Autodesk Fusion 360 part; units mm, degrees
(part 6 of 8)
  spline S170 degree 5 poles (-253.8232, -300.3539) (-253.7673, -300.4279) (-253.6554, -300.5759) (-253.4871, -300.7975) (-253.2622, -301.0921) (-252.9798, -301.4591) (-252.6964, -301.8248) (-252.4118, -302.1892) (-252.1261, -302.5523) (-251.8392, -302.914) (-251.5513, -303.2744) (-251.2621, -303.6334) (-250.9719, -303.9911) (-250.6805, -304.3474) (-250.388, -304.7023) (-250.0943, -305.0558) (-249.7994, -305.4078) (-249.5034, -305.7584) (-249.2062, -306.1076) (-248.9079, -306.4553) (-248.6083, -306.8015) (-248.3076, -307.1462) (-248.0057, -307.4895) (-247.7026, -307.8312) (-247.3983, -308.1713) (-247.0928, -308.5099) (-246.7861, -308.8469) (-246.4782, -309.1823) (-246.1691, -309.5161) (-245.8587, -309.8483) (-245.5471, -310.1788) (-245.2342, -310.5077) (-244.9201, -310.8348) (-244.6048, -311.1603) (-244.2881, -311.484) (-243.9702, -311.8059) (-243.651, -312.1261) (-243.3305, -312.4444) (-243.0087, -312.7609) (-242.6855, -313.0755) (-242.361, -313.3882) (-242.0352, -313.699) (-241.7081, -314.0079) (-241.3795, -314.3147) (-241.0496, -314.6196) (-240.7183, -314.9223) (-240.3856, -315.223) (-240.0514, -315.5215) (-239.7157, -315.8178) (-239.3786, -316.1118) (-239.04, -316.4036) (-238.6999, -316.6931) (-238.3583, -316.9802) (-238.0151, -317.2649) (-237.6704, -317.5471) (-237.324, -317.8267) (-236.9759, -318.1036) (-236.626, -318.3775) (-236.2744, -318.6485) (-235.921, -318.9166) (-235.5658, -319.1817) (-235.2088, -319.4439) (-234.85, -319.703) (-234.525, -319.9335) (-234.2708, -320.1107) (-234.0884, -320.236) (-233.9786, -320.3108) (-233.9417, -320.3358) knots -1 -1 -1 -1 -1 -1 -0.98571429 -0.97142857 -0.95714286 -0.94285714 -0.92857143 -0.91428571 -0.9 -0.88571429 -0.87142857 -0.85714286 -0.84285714 -0.82857143 -0.81428571 -0.8 -0.78571429 -0.77142857 -0.75714286 -0.74285714 -0.72857143 -0.71428571 -0.7 -0.68571429 -0.67142857 -0.65714286 -0.64285714 -0.62857143 -0.61428571 -0.6 -0.58571429 -0.57142857 -0.55714286 -0.54285714 -0.52857143 -0.51428571 -0.5 -0.48571429 -0.47142857 -0.45714286 -0.44285714 -0.42857143 -0.41428571 -0.4 -0.38571429 -0.37142857 -0.35714286 -0.34285714 -0.32857143 -0.31428571 -0.3 -0.28571429 -0.27142857 -0.25714286 -0.24285714 -0.22857143 -0.21428571 -0.2 -0.18571429 -0.17142857 -0.15714286 -0.14285714 -0.12857143 -0.11428571 -0.10707295 -0.10707295 -0.10707295 -0.10707295 -0.10707295 -0.10707295
  spline S171 degree 3 poles (-233.3933, -322.3173) (-233.3063, -322.1298) (-233.2568, -321.9271) (-233.2382, -321.5141) (-233.2694, -321.3077) (-233.3956, -320.956) (-233.4764, -320.8087) (-233.681, -320.5447) (-233.8036, -320.4296) (-233.9417, -320.3358) knots 0 0 0 0 0.062015 0.062015 0.12403 0.12403 0.174133 0.174133 0.224236 0.224236 0.224236 0.224236
  arc A86 (-233.3933, -322.3173) -> (-236.8029, -329.9753) centre (11.949, -436.1388) ccw
  spline S172 degree 3 poles (-238.6424, -330.8936) (-238.4416, -330.943) (-238.2332, -330.9527) (-237.8243, -330.8918) (-237.6277, -330.8216) (-237.3067, -330.6303) (-237.1776, -330.5227) (-236.9578, -330.2712) (-236.8684, -330.1289) (-236.8029, -329.9753) knots 0 0 0 0 0.062015 0.062015 0.12403 0.12403 0.174133 0.174133 0.224236 0.224236 0.224236 0.224236
  spline S173 degree 5 poles (-238.6424, -330.8936) (-238.6857, -330.883) (-238.8147, -330.8514) (-239.0299, -330.7997) (-239.3316, -330.7294) (-239.7204, -330.6421) (-240.153, -330.5488) (-240.5867, -330.459) (-241.0214, -330.3724) (-241.4571, -330.2891) (-241.8938, -330.2092) (-242.3315, -330.1325) (-242.7701, -330.059) (-243.2097, -329.9887) (-243.6501, -329.9213) (-244.0913, -329.8569) (-244.5333, -329.7951) (-244.976, -329.7361) (-245.4194, -329.6797) (-245.8635, -329.6259) (-246.3083, -329.5747) (-246.7537, -329.5261) (-247.1998, -329.48) (-247.6465, -329.4363) (-248.0938, -329.3952) (-248.5416, -329.3563) (-248.9901, -329.3199) (-249.4391, -329.2857) (-249.8886, -329.2538) (-250.3386, -329.2242) (-250.7891, -329.1968) (-251.2402, -329.1716) (-251.6917, -329.1486) (-252.1437, -329.1278) (-252.5961, -329.1091) (-253.049, -329.0925) (-253.5023, -329.078) (-253.956, -329.0655) (-254.4101, -329.0551) (-254.8647, -329.0467) (-255.3196, -329.0403) (-255.7749, -329.0359) (-256.2306, -329.0335) (-256.6866, -329.0331) (-257.143, -329.0345) (-257.5997, -329.0379) (-258.0568, -329.0432) (-258.5142, -329.0504) (-258.9719, -329.0595) (-259.4299, -329.0705) (-259.8883, -329.0832) (-260.3469, -329.0979) (-260.8058, -329.1143) (-261.265, -329.1326) (-261.7245, -329.1526) (-262.1843, -329.1745) (-262.6443, -329.1981) (-263.1045, -329.2235) (-263.5651, -329.2507) (-264.0258, -329.2795) (-264.4868, -329.3102) (-264.948, -329.3425) (-265.4094, -329.3765) (-265.8711, -329.4123) (-266.2406, -329.4423) (-266.5178, -329.4655) (-266.7027, -329.4813) (-266.7951, -329.4893) knots 0.10707295 0.10707295 0.10707295 0.10707295 0.10707295 0.10707295 0.11428571 0.12857143 0.14285714 0.15714286 0.17142857 0.18571429 0.2 0.21428571 0.22857143 0.24285714 0.25714286 0.27142857 0.28571429 0.3 0.31428571 0.32857143 0.34285714 0.35714286 0.37142857 0.38571429 0.4 0.41428571 0.42857143 0.44285714 0.45714286 0.47142857 0.48571429 0.5 0.51428571 0.52857143 0.54285714 0.55714286 0.57142857 0.58571429 0.6 0.61428571 0.62857143 0.64285714 0.65714286 0.67142857 0.68571429 0.7 0.71428571 0.72857143 0.74285714 0.75714286 0.77142857 0.78571429 0.8 0.81428571 0.82857143 0.84285714 0.85714286 0.87142857 0.88571429 0.9 0.91428571 0.92857143 0.94285714 0.95714286 0.97142857 0.98571429 1 1 1 1 1 1
  arc A87 (-266.7951, -329.4893) -> (-270.1343, -338.6637) centre (11.949, -436.1388) ccw
  spline S174 degree 5 poles (-270.1343, -338.6637) (-270.0687, -338.7292) (-269.9372, -338.8602) (-269.7398, -339.0562) (-269.476, -339.3167) (-269.1453, -339.6408) (-268.8137, -339.9635) (-268.4812, -340.2847) (-268.1477, -340.6045) (-267.8134, -340.9228) (-267.478, -341.2396) (-267.1418, -341.5549) (-266.8046, -341.8687) (-266.4664, -342.1809) (-266.1273, -342.4917) (-265.7873, -342.8008) (-265.4463, -343.1084) (-265.1044, -343.4144) (-264.7615, -343.7188) (-264.4177, -344.0216) (-264.0729, -344.3228) (-263.7271, -344.6223) (-263.3804, -344.9202) (-263.0327, -345.2164) (-262.684, -345.5108) (-262.3344, -345.8036) (-261.9837, -346.0947) (-261.6321, -346.384) (-261.2796, -346.6715) (-260.926, -346.9573) (-260.5714, -347.2412) (-260.2158, -347.5233) (-259.8592, -347.8035) (-259.5016, -348.0819) (-259.143, -348.3584) (-258.7834, -348.633) (-258.4227, -348.9056) (-258.061, -349.1762) (-257.6983, -349.4448) (-257.3345, -349.7114) (-256.9697, -349.9759) (-256.6038, -350.2384) (-256.2368, -350.4987) (-255.8688, -350.7568) (-255.4997, -351.0128) (-255.1294, -351.2665) (-254.7581, -351.5179) (-254.3856, -351.767) (-254.012, -352.0137) (-253.6372, -352.2579) (-253.2613, -352.4998) (-252.8842, -352.7391) (-252.506, -352.9759) (-252.1265, -353.2101) (-251.7458, -353.4416) (-251.3639, -353.6702) (-250.9807, -353.8959) (-250.5961, -354.1185) (-250.2102, -354.338) (-249.8229, -354.5542) (-249.4342, -354.7673) (-249.0442, -354.9773) (-248.6529, -355.1839) (-248.2989, -355.367) (-248.0226, -355.507) (-247.8246, -355.6057) (-247.7054, -355.6645) (-247.6654, -355.6842) knots -1 -1 -1 -1 -1 -1 -0.98571429 -0.97142857 -0.95714286 -0.94285714 -0.92857143 -0.91428571 -0.9 -0.88571429 -0.87142857 -0.85714286 -0.84285714 -0.82857143 -0.81428571 -0.8 -0.78571429 -0.77142857 -0.75714286 -0.74285714 -0.72857143 -0.71428571 -0.7 -0.68571429 -0.67142857 -0.65714286 -0.64285714 -0.62857143 -0.61428571 -0.6 -0.58571429 -0.57142857 -0.55714286 -0.54285714 -0.52857143 -0.51428571 -0.5 -0.48571429 -0.47142857 -0.45714286 -0.44285714 -0.42857143 -0.41428571 -0.4 -0.38571429 -0.37142857 -0.35714286 -0.34285714 -0.32857143 -0.31428571 -0.3 -0.28571429 -0.27142857 -0.25714286 -0.24285714 -0.22857143 -0.21428571 -0.2 -0.18571429 -0.17142857 -0.15714286 -0.14285714 -0.12857143 -0.11428571 -0.10707295 -0.10707295 -0.10707295 -0.10707295 -0.10707295 -0.10707295
  spline S175 degree 3 poles (-246.8466, -357.5701) (-246.7865, -357.3723) (-246.7657, -357.1647) (-246.8047, -356.7531) (-246.8643, -356.5531) (-247.0382, -356.2223) (-247.1388, -356.0877) (-247.3782, -355.8547) (-247.5155, -355.7579) (-247.6654, -355.6842) knots 0 0 0 0 0.062015 0.062015 0.12403 0.12403 0.174133 0.174133 0.224236 0.224236 0.224236 0.224236
  arc A88 (-246.8466, -357.5701) -> (-249.1571, -365.628) centre (11.949, -436.1388) ccw
  spline S176 degree 3 poles (-250.8509, -366.7934) (-250.6453, -366.8144) (-250.4375, -366.795) (-250.0411, -366.6777) (-249.8562, -366.5809) (-249.5649, -366.3468) (-249.4521, -366.2222) (-249.2694, -365.9426) (-249.2007, -365.7892) (-249.1571, -365.628) knots 0 0 0 0 0.062015 0.062015 0.12403 0.12403 0.174133 0.174133 0.224236 0.224236 0.224236 0.224236
  spline S177 degree 5 poles (-250.8509, -366.7934) (-250.8953, -366.7889) (-251.0275, -366.7756) (-251.2477, -366.7544) (-251.5563, -366.7267) (-251.9534, -366.6944) (-252.3948, -366.6623) (-252.8368, -366.6336) (-253.2794, -366.6084) (-253.7224, -366.5866) (-254.166, -366.5682) (-254.6101, -366.5531) (-255.0547, -366.5415) (-255.4997, -366.533) (-255.9453, -366.5276) (-256.3911, -366.5251) (-256.8374, -366.5255) (-257.284, -366.5286) (-257.7309, -366.5345) (-258.1782, -366.543) (-258.6258, -366.5542) (-259.0736, -366.5681) (-259.5218, -366.5845) (-259.9702, -366.6035) (-260.4189, -366.6249) (-260.8678, -366.6488) (-261.317, -366.6751) (-261.7663, -366.7038) (-262.2159, -366.7348) (-262.6657, -366.7681) (-263.1156, -366.8037) (-263.5658, -366.8415) (-264.0161, -366.8816) (-264.4666, -366.9238) (-264.9172, -366.9683) (-265.368, -367.0148) (-265.8189, -367.0636) (-266.2699, -367.1144) (-266.7211, -367.1673) (-267.1724, -367.2222) (-267.6238, -367.2792) (-268.0752, -367.3382) (-268.5268, -367.3993) (-268.9785, -367.4623) (-269.4302, -367.5272) (-269.882, -367.5942) (-270.3339, -367.663) (-270.7859, -367.7338) (-271.2379, -367.8065) (-271.6899, -367.8811) (-272.142, -367.9575) (-272.5941, -368.0358) (-273.0463, -368.116) (-273.4985, -368.198) (-273.9507, -368.2818) (-274.403, -368.3674) (-274.8552, -368.4549) (-275.3075, -368.5441) (-275.7597, -368.635) (-276.212, -368.7278) (-276.6642, -368.8222) (-277.1164, -368.9184) (-277.5686, -369.0164) (-278.0208, -369.116) (-278.3826, -369.1971) (-278.6539, -369.2587) (-278.8347, -369.3001) (-278.9252, -369.3209) knots 0.10707295 0.10707295 0.10707295 0.10707295 0.10707295 0.10707295 0.11428571 0.12857143 0.14285714 0.15714286 0.17142857 0.18571429 0.2 0.21428571 0.22857143 0.24285714 0.25714286 0.27142857 0.28571429 0.3 0.31428571 0.32857143 0.34285714 0.35714286 0.37142857 0.38571429 0.4 0.41428571 0.42857143 0.44285714 0.45714286 0.47142857 0.48571429 0.5 0.51428571 0.52857143 0.54285714 0.55714286 0.57142857 0.58571429 0.6 0.61428571 0.62857143 0.64285714 0.65714286 0.67142857 0.68571429 0.7 0.71428571 0.72857143 0.74285714 0.75714286 0.77142857 0.78571429 0.8 0.81428571 0.82857143 0.84285714 0.85714286 0.87142857 0.88571429 0.9 0.91428571 0.92857143 0.94285714 0.95714286 0.97142857 0.98571429 1 1 1 1 1 1
  arc A89 (-278.9252, -369.3209) -> (-280.955, -378.8707) centre (11.949, -436.1388) ccw
  spline S178 degree 5 poles (-280.955, -378.8707) (-280.8809, -378.9265) (-280.7325, -379.0379) (-280.5097, -379.2045) (-280.2122, -379.4257) (-279.8397, -379.7007) (-279.4664, -379.9741) (-279.0924, -380.2459) (-278.7177, -380.5161) (-278.3422, -380.7848) (-277.9661, -381.0519) (-277.5892, -381.3173) (-277.2116, -381.5811) (-276.8333, -381.8433) (-276.4543, -382.1038) (-276.0745, -382.3626) (-275.6941, -382.6197) (-275.3129, -382.8752) (-274.9309, -383.1289) (-274.5483, -383.3809) (-274.165, -383.6311) (-273.7809, -383.8796) (-273.3961, -384.1263) (-273.0105, -384.3713) (-272.6243, -384.6144) (-272.2373, -384.8556) (-271.8496, -385.0951) (-271.4611, -385.3326) (-271.0719, -385.5683) (-270.682, -385.802) (-270.2914, -386.0338) (-269.9, -386.2637) (-269.5079, -386.4916) (-269.115, -386.7175) (-268.7214, -386.9414) (-268.3271, -387.1632) (-267.932, -387.383) (-267.5362, -387.6007) (-267.1396, -387.8162) (-266.7422, -388.0295) (-266.3441, -388.2407) (-265.9453, -388.4497) (-265.5457, -388.6564) (-265.1453, -388.8608) (-264.7441, -389.0629) (-264.3422, -389.2626) (-263.9394, -389.4599) (-263.5359, -389.6547) (-263.1316, -389.847) (-262.7265, -390.0367) (-262.3206, -390.2239) (-261.9139, -390.4084) (-261.5063, -390.5902) (-261.098, -390.7693) (-260.6888, -390.9456) (-260.2788, -391.1189) (-259.8679, -391.289) (-259.456, -391.456) (-259.0433, -391.6196) (-258.6297, -391.7798) (-258.2152, -391.9368) (-257.7998, -392.0904) (-257.3834, -392.2406) (-257.0075, -392.3726) (-256.7143, -392.4728) (-256.5045, -392.543) (-256.3783, -392.5846) (-256.336, -392.5985) knots -1 -1 -1 -1 -1 -1 -0.98571429 -0.97142857 -0.95714286 -0.94285714 -0.92857143 -0.91428571 -0.9 -0.88571429 -0.87142857 -0.85714286 -0.84285714 -0.82857143 -0.81428571 -0.8 -0.78571429 -0.77142857 -0.75714286 -0.74285714 -0.72857143 -0.71428571 -0.7 -0.68571429 -0.67142857 -0.65714286 -0.64285714 -0.62857143 -0.61428571 -0.6 -0.58571429 -0.57142857 -0.55714286 -0.54285714 -0.52857143 -0.51428571 -0.5 -0.48571429 -0.47142857 -0.45714286 -0.44285714 -0.42857143 -0.41428571 -0.4 -0.38571429 -0.37142857 -0.35714286 -0.34285714 -0.32857143 -0.31428571 -0.3 -0.28571429 -0.27142857 -0.25714286 -0.24285714 -0.22857143 -0.21428571 -0.2 -0.18571429 -0.17142857 -0.15714286 -0.14285714 -0.12857143 -0.11428571 -0.10707295 -0.10707295 -0.10707295 -0.10707295 -0.10707295 -0.10707295
  spline S179 degree 3 poles (-255.2626, -394.3521) (-255.2307, -394.1479) (-255.2389, -393.9394) (-255.3349, -393.5372) (-255.4217, -393.3474) (-255.64, -393.0441) (-255.7583, -392.9248) (-256.0278, -392.7274) (-256.1773, -392.6506) (-256.336, -392.5985) knots 0 0 0 0 0.062015 0.062015 0.12403 0.12403 0.174133 0.174133 0.224236 0.224236 0.224236 0.224236
  circle A90 centre (11.949, -436.1388) radius 6.35
  circle A91 centre (11.949, -436.1388) radius 6.35
  constraint concentric A0 A91
extrude "Extrude1''" add sketch "Sketch1 (3)" along normal mid plane 100 separate body contours A90 A91 makes body 3 in component "Component"
sketch "Sketch2 (3)" plane through (0, 0, 12.7) normal (0, 0, 1) x (-1, 0, 0)
  arc A0 (-132.9976, 25.7536) -> (-134.3966, 15.1274) centre (2.1352, 2.5578) ccw
  arc A1 (-136.1046, 13.6905) -> (-134.3966, 15.1274) centre (-135.9774, 15.2729) ccw
  line L0 (-136.1046, 13.6905) -> (-140.6118, 14.0529)
  spline S0 degree 5 poles (-140.6118, 14.0529) (-140.6765, 14.0581) (-140.806, 14.0668) (-141.0002, 14.0751) (-141.2594, 14.0767) (-141.5836, 14.066) (-141.908, 14.0461) (-142.2326, 14.0206) (-142.5571, 13.9921) (-142.8817, 13.9616) (-143.2063, 13.9289) (-143.5308, 13.8933) (-143.8552, 13.8539) (-144.1796, 13.81) (-144.5039, 13.7617) (-144.828, 13.7094) (-145.1521, 13.6535) (-145.476, 13.5948) (-145.7998, 13.5335) (-146.1234, 13.4699) (-146.4468, 13.4038) (-146.7701, 13.3352) (-147.0932, 13.264) (-147.4161, 13.19) (-147.7389, 13.1133) (-148.0614, 13.034) (-148.3837, 12.9523) (-148.7058, 12.8683) (-149.0277, 12.782) (-149.3494, 12.6936) (-149.6708, 12.6029) (-149.992, 12.5101) (-150.313, 12.4152) (-150.6337, 12.318) (-150.9541, 12.2188) (-151.2743, 12.1174) (-151.5943, 12.014) (-151.9139, 11.9086) (-152.2333, 11.8012) (-152.5524, 11.6919) (-152.8713, 11.5806) (-153.1898, 11.4675) (-153.5081, 11.3524) (-153.8261, 11.2354) (-154.1437, 11.1166) (-154.4611, 10.996) (-154.7782, 10.8735) (-155.0949, 10.7492) (-155.4114, 10.6232) (-155.7275, 10.4954) (-156.0433, 10.3658) (-156.3588, 10.2345) (-156.6739, 10.1015) (-156.9887, 9.9668) (-157.3032, 9.8305) (-157.6173, 9.6924) (-157.9311, 9.5527) (-158.2446, 9.4113) (-158.5577, 9.2683) (-158.8704, 9.1237) (-159.1828, 8.9774) (-159.4948, 8.8296) (-159.8065, 8.6802) (-160.1178, 8.5292) (-160.4287, 8.3767) (-160.7392, 8.2226) (-161.0494, 8.0669) (-161.3592, 7.9098) (-161.6686, 7.7511) (-161.9776, 7.5909) (-162.2863, 7.4292) (-162.5328, 7.2987) (-162.7176, 7.2001) (-162.8407, 7.1341) (-162.9023, 7.101) knots 0 0 0 0 0 0 0.01428571 0.02857143 0.04285714 0.05714286 0.07142857 0.08571429 0.1 0.11428571 0.12857143 0.14285714 0.15714286 0.17142857 0.18571429 0.2 0.21428571 0.22857143 0.24285714 0.25714286 0.27142857 0.28571429 0.3 0.31428571 0.32857143 0.34285714 0.35714286 0.37142857 0.38571429 0.4 0.41428571 0.42857143 0.44285714 0.45714286 0.47142857 0.48571429 0.5 0.51428571 0.52857143 0.54285714 0.55714286 0.57142857 0.58571429 0.6 0.61428571 0.62857143 0.64285714 0.65714286 0.67142857 0.68571429 0.7 0.71428571 0.72857143 0.74285714 0.75714286 0.77142857 0.78571429 0.8 0.81428571 0.82857143 0.84285714 0.85714286 0.87142857 0.88571429 0.9 0.91428571 0.92857143 0.94285714 0.95714286 0.97142857 0.98571429 1 1 1 1 1 1
  arc A2 (-162.9023, 7.101) -> (-162.9023, -1.9854) centre (2.1352, 2.5578) ccw
  spline S1 degree 5 poles (-162.9023, -1.9854) (-162.8407, -2.0185) (-162.7176, -2.0845) (-162.5328, -2.1831) (-162.2863, -2.3136) (-161.9776, -2.4753) (-161.6686, -2.6355) (-161.3592, -2.7942) (-161.0494, -2.9513) (-160.7392, -3.107) (-160.4287, -3.2611) (-160.1178, -3.4136) (-159.8065, -3.5646) (-159.4948, -3.714) (-159.1828, -3.8618) (-158.8704, -4.0081) (-158.5577, -4.1527) (-158.2446, -4.2957) (-157.9311, -4.4371) (-157.6173, -4.5768) (-157.3032, -4.7148) (-156.9887, -4.8512) (-156.6739, -4.9859) (-156.3588, -5.1189) (-156.0433, -5.2502) (-155.7275, -5.3798) (-155.4114, -5.5076) (-155.0949, -5.6336) (-154.7782, -5.7579) (-154.4611, -5.8804) (-154.1437, -6.001) (-153.8261, -6.1198) (-153.5081, -6.2368) (-153.1898, -6.3518) (-152.8713, -6.465) (-152.5524, -6.5763) (-152.2333, -6.6856) (-151.9139, -6.793) (-151.5943, -6.8984) (-151.2743, -7.0018) (-150.9541, -7.1032) (-150.6337, -7.2024) (-150.313, -7.2996) (-149.992, -7.3945) (-149.6708, -7.4873) (-149.3494, -7.5779) (-149.0277, -7.6664) (-148.7058, -7.7527) (-148.3837, -7.8367) (-148.0614, -7.9184) (-147.7389, -7.9977) (-147.4161, -8.0744) (-147.0932, -8.1484) (-146.7701, -8.2196) (-146.4468, -8.2882) (-146.1234, -8.3543) (-145.7998, -8.4179) (-145.476, -8.4792) (-145.1521, -8.5379) (-144.828, -8.5938) (-144.5039, -8.6461) (-144.1796, -8.6944) (-143.8552, -8.7383) (-143.5308, -8.7777) (-143.2063, -8.8133) (-142.8817, -8.846) (-142.5571, -8.8765) (-142.2326, -8.905) (-141.908, -8.9305) (-141.5836, -8.9504) (-141.2594, -8.9611) (-141.0002, -8.9595) (-140.806, -8.9512) (-140.6765, -8.9425) (-140.6118, -8.9373) knots -1 -1 -1 -1 -1 -1 -0.98571429 -0.97142857 -0.95714286 -0.94285714 -0.92857143 -0.91428571 -0.9 -0.88571429 -0.87142857 -0.85714286 -0.84285714 -0.82857143 -0.81428571 -0.8 -0.78571429 -0.77142857 -0.75714286 -0.74285714 -0.72857143 -0.71428571 -0.7 -0.68571429 -0.67142857 -0.65714286 -0.64285714 -0.62857143 -0.61428571 -0.6 -0.58571429 -0.57142857 -0.55714286 -0.54285714 -0.52857143 -0.51428571 -0.5 -0.48571429 -0.47142857 -0.45714286 -0.44285714 -0.42857143 -0.41428571 -0.4 -0.38571429 -0.37142857 -0.35714286 -0.34285714 -0.32857143 -0.31428571 -0.3 -0.28571429 -0.27142857 -0.25714286 -0.24285714 -0.22857143 -0.21428571 -0.2 -0.18571429 -0.17142857 -0.15714286 -0.14285714 -0.12857143 -0.11428571 -0.1 -0.08571429 -0.07142857 -0.05714286 -0.04285714 -0.02857143 -0.01428571 0 0 0 0 0 0
  line L1 (-140.6118, -8.9373) -> (-136.1046, -8.5749)
  arc A3 (-134.3966, -10.0118) -> (-136.1046, -8.5749) centre (-135.9774, -10.1573) ccw
  arc A4 (-134.3966, -10.0118) -> (-132.9976, -20.6379) centre (2.1352, 2.5578) ccw
  arc A5 (-134.2756, -22.4679) -> (-132.9976, -20.6379) centre (-134.5623, -20.9065) ccw
  line L2 (-134.2756, -22.4679) -> (-138.723, -23.2845)
  spline S2 degree 5 poles (-138.723, -23.2845) (-138.7868, -23.2962) (-138.9141, -23.3212) (-139.1039, -23.3635) (-139.3546, -23.4291) (-139.665, -23.5233) (-139.9733, -23.6265) (-140.2801, -23.7351) (-140.5863, -23.8466) (-140.8919, -23.9601) (-141.1969, -24.0757) (-141.5012, -24.1941) (-141.8044, -24.3161) (-142.1063, -24.4424) (-142.4071, -24.573) (-142.7066, -24.7075) (-143.0052, -24.8453) (-143.3028, -24.9859) (-143.5997, -25.1289) (-143.8958, -25.2741) (-144.1912, -25.4216) (-144.4857, -25.5715) (-144.7794, -25.724) (-145.0721, -25.879) (-145.364, -26.0366) (-145.655, -26.1967) (-145.9452, -26.359) (-146.2346, -26.5236) (-146.5232, -26.6902) (-146.811, -26.8589) (-147.098, -27.0296) (-147.3843, -27.2024) (-147.6697, -27.3772) (-147.9543, -27.554) (-148.2382, -27.7329) (-148.5212, -27.9136) (-148.8035, -28.0963) (-149.085, -28.2809) (-149.3657, -28.4673) (-149.6457, -28.6555) (-149.9248, -28.8455) (-150.2032, -29.0372) (-150.4809, -29.2307) (-150.7577, -29.426) (-151.0338, -29.623) (-151.3092, -29.8217) (-151.5837, -30.022) (-151.8575, -30.224) (-152.1306, -30.4277) (-152.4028, -30.633) (-152.6743, -30.8398) (-152.9451, -31.0483) (-153.2151, -31.2583) (-153.4843, -31.4699) (-153.7528, -31.6831) (-154.0205, -31.8977) (-154.2874, -32.1139) (-154.5536, -32.3316) (-154.819, -32.5507) (-155.0836, -32.7714) (-155.3475, -32.9935) (-155.6107, -33.217) (-155.873, -33.442) (-156.1346, -33.6684) (-156.3955, -33.8962) (-156.6556, -34.1255) (-156.9149, -34.3561) (-157.1735, -34.5881) (-157.4312, -34.8214) (-157.6883, -35.0561) (-157.9445, -35.2922) (-158.1489, -35.4821) (-158.3019, -35.6252) (-158.4037, -35.7208) (-158.4546, -35.7687) knots 0 0 0 0 0 0 0.01428571 0.02857143 0.04285714 0.05714286 0.07142857 0.08571429 0.1 0.11428571 0.12857143 0.14285714 0.15714286 0.17142857 0.18571429 0.2 0.21428571 0.22857143 0.24285714 0.25714286 0.27142857 0.28571429 0.3 0.31428571 0.32857143 0.34285714 0.35714286 0.37142857 0.38571429 0.4 0.41428571 0.42857143 0.44285714 0.45714286 0.47142857 0.48571429 0.5 0.51428571 0.52857143 0.54285714 0.55714286 0.57142857 0.58571429 0.6 0.61428571 0.62857143 0.64285714 0.65714286 0.67142857 0.68571429 0.7 0.71428571 0.72857143 0.74285714 0.75714286 0.77142857 0.78571429 0.8 0.81428571 0.82857143 0.84285714 0.85714286 0.87142857 0.88571429 0.9 0.91428571 0.92857143 0.94285714 0.95714286 0.97142857 0.98571429 1 1 1 1 1 1
  arc A6 (-158.4546, -35.7687) -> (-156.1029, -44.5454) centre (2.1352, 2.5578) ccw
  spline S3 degree 5 poles (-156.1029, -44.5454) (-156.0349, -44.5614) (-155.8989, -44.5934) (-155.6949, -44.6408) (-155.4229, -44.703) (-155.0829, -44.7793) (-154.743, -44.8541) (-154.4031, -44.9273) (-154.0632, -44.9989) (-153.7233, -45.069) (-153.3834, -45.1374) (-153.0436, -45.2043) (-152.7038, -45.2696) (-152.3641, -45.3332) (-152.0245, -45.3953) (-151.6849, -45.4557) (-151.3454, -45.5144) (-151.0059, -45.5715) (-150.6666, -45.6269) (-150.3273, -45.6807) (-149.9882, -45.7327) (-149.6491, -45.7831) (-149.3101, -45.8317) (-148.9713, -45.8786) (-148.6326, -45.9238) (-148.294, -45.9672) (-147.9556, -46.0088) (-147.6173, -46.0487) (-147.2792, -46.0867) (-146.9413, -46.1229) (-146.6035, -46.1573) (-146.2659, -46.1899) (-145.9285, -46.2206) (-145.5913, -46.2493) (-145.2543, -46.2762) (-144.9175, -46.3012) (-144.581, -46.3242) (-144.2447, -46.3452) (-143.9086, -46.3643) (-143.5728, -46.3814) (-143.2373, -46.3964) (-142.9021, -46.4094) (-142.5671, -46.4202) (-142.2325, -46.4288) (-141.8983, -46.4353) (-141.5643, -46.4397) (-141.2307, -46.4419) (-140.8975, -46.4419) (-140.5646, -46.4397) (-140.2321, -46.4352) (-139.9001, -46.4283) (-139.5685, -46.4189) (-139.2374, -46.4067) (-138.9069, -46.3919) (-138.5769, -46.3745) (-138.2473, -46.3546) (-137.9183, -46.3323) (-137.5897, -46.3077) (-137.2616, -46.2806) (-136.9341, -46.2507) (-136.6075, -46.2174) (-136.2817, -46.1801) (-135.9571, -46.1385) (-135.6335, -46.0926) (-135.3108, -46.043) (-134.9889, -45.9906) (-134.6674, -45.936) (-134.3466, -45.8796) (-134.0265, -45.8202) (-133.708, -45.7554) (-133.392, -45.6818) (-133.1421, -45.6132) (-132.9566, -45.555) (-132.8339, -45.513) (-132.7727, -45.4913) knots -1 -1 -1 -1 -1 -1 -0.98571429 -0.97142857 -0.95714286 -0.94285714 -0.92857143 -0.91428571 -0.9 -0.88571429 -0.87142857 -0.85714286 -0.84285714 -0.82857143 -0.81428571 -0.8 -0.78571429 -0.77142857 -0.75714286 -0.74285714 -0.72857143 -0.71428571 -0.7 -0.68571429 -0.67142857 -0.65714286 -0.64285714 -0.62857143 -0.61428571 -0.6 -0.58571429 -0.57142857 -0.55714286 -0.54285714 -0.52857143 -0.51428571 -0.5 -0.48571429 -0.47142857 -0.45714286 -0.44285714 -0.42857143 -0.41428571 -0.4 -0.38571429 -0.37142857 -0.35714286 -0.34285714 -0.32857143 -0.31428571 -0.3 -0.28571429 -0.27142857 -0.25714286 -0.24285714 -0.22857143 -0.21428571 -0.2 -0.18571429 -0.17142857 -0.15714286 -0.14285714 -0.12857143 -0.11428571 -0.1 -0.08571429 -0.07142857 -0.05714286 -0.04285714 -0.02857143 -0.01428571 0 0 0 0 0 0
  line L3 (-132.7727, -45.4913) -> (-128.5129, -43.9747)
  arc A7 (-126.4911, -44.9205) -> (-128.5129, -43.9747) centre (-127.9804, -45.4702) ccw
  arc A8 (-126.4911, -44.9205) -> (-122.3896, -54.8225) centre (2.1352, 2.5578) ccw
  arc A9 (-123.1504, -56.9209) -> (-122.3896, -54.8225) centre (-123.8314, -55.4869) ccw
  line L4 (-123.1504, -56.9209) -> (-127.2349, -58.8607)
  spline S4 degree 5 poles (-127.2349, -58.8607) (-127.2935, -58.8885) (-127.41, -58.9457) (-127.5823, -59.0357) (-127.8076, -59.1639) (-128.083, -59.3353) (-128.354, -59.5147) (-128.6223, -59.699) (-128.8892, -59.886) (-129.155, -60.0747) (-129.4198, -60.2653) (-129.683, -60.4584) (-129.9443, -60.6547) (-130.2032, -60.8549) (-130.4599, -61.0588) (-130.7145, -61.2663) (-130.9672, -61.4767) (-131.2183, -61.6895) (-131.4681, -61.9045) (-131.7165, -62.1214) (-131.9636, -62.3403) (-132.2093, -62.5613) (-132.4535, -62.7846) (-132.6962, -63.0101) (-132.9373, -63.2379) (-133.177, -63.4678) (-133.4153, -63.6998) (-133.6522, -63.9336) (-133.8878, -64.1692) (-134.1222, -64.4067) (-134.3552, -64.6459) (-134.587, -64.8868) (-134.8175, -65.1296) (-135.0466, -65.374) (-135.2745, -65.6202) (-135.5011, -65.8681) (-135.7265, -66.1176) (-135.9506, -66.3687) (-136.1736, -66.6214) (-136.3953, -66.8757) (-136.6157, -67.1315) (-136.835, -67.3887) (-137.0531, -67.6475) (-137.27, -67.9078) (-137.4857, -68.1695) (-137.7003, -68.4327) (-137.9136, -68.6973) (-138.1258, -68.9633) (-138.3368, -69.2307) (-138.5467, -69.4994) (-138.7554, -69.7695) (-138.963, -70.0409) (-139.1694, -70.3137) (-139.3747, -70.5877) (-139.5788, -70.8631) (-139.7818, -71.1397) (-139.9837, -71.4176) (-140.1845, -71.6968) (-140.3841, -71.9772) (-140.5827, -72.2588) (-140.7801, -72.5416) (-140.9764, -72.8257) (-141.1716, -73.1109) (-141.3657, -73.3973) (-141.5587, -73.6849) (-141.7506, -73.9736) (-141.9414, -74.2635) (-142.1311, -74.5545) (-142.3197, -74.8466) (-142.5072, -75.1398) (-142.6937, -75.4342) (-142.8419, -75.6705) (-142.9527, -75.8483) (-143.0263, -75.967) (-143.063, -76.0264) knots 0 0 0 0 0 0 0.01428571 0.02857143 0.04285714 0.05714286 0.07142857 0.08571429 0.1 0.11428571 0.12857143 0.14285714 0.15714286 0.17142857 0.18571429 0.2 0.21428571 0.22857143 0.24285714 0.25714286 0.27142857 0.28571429 0.3 0.31428571 0.32857143 0.34285714 0.35714286 0.37142857 0.38571429 0.4 0.41428571 0.42857143 0.44285714 0.45714286 0.47142857 0.48571429 0.5 0.51428571 0.52857143 0.54285714 0.55714286 0.57142857 0.58571429 0.6 0.61428571 0.62857143 0.64285714 0.65714286 0.67142857 0.68571429 0.7 0.71428571 0.72857143 0.74285714 0.75714286 0.77142857 0.78571429 0.8 0.81428571 0.82857143 0.84285714 0.85714286 0.87142857 0.88571429 0.9 0.91428571 0.92857143 0.94285714 0.95714286 0.97142857 0.98571429 1 1 1 1 1 1
  arc A10 (-143.063, -76.0264) -> (-138.5198, -83.8954) centre (2.1352, 2.5578) ccw
  spline S5 degree 5 poles (-138.5198, -83.8954) (-138.45, -83.8933) (-138.3104, -83.889) (-138.1011, -83.8819) (-137.8222, -83.8717) (-137.4741, -83.8574) (-137.1264, -83.8416) (-136.7791, -83.8244) (-136.4322, -83.8056) (-136.0858, -83.7853) (-135.7398, -83.7634) (-135.3943, -83.7401) (-135.0492, -83.7152) (-134.7046, -83.6888) (-134.3604, -83.6608) (-134.0168, -83.6312) (-133.6736, -83.6001) (-133.331, -83.5674) (-132.9889, -83.5331) (-132.6472, -83.4972) (-132.3062, -83.4597) (-131.9656, -83.4206) (-131.6256, -83.3798) (-131.2862, -83.3374) (-130.9474, -83.2934) (-130.6091, -83.2477) (-130.2714, -83.2003) (-129.9344, -83.1513) (-129.5979, -83.1005) (-129.2621, -83.048) (-128.9269, -82.9938) (-128.5924, -82.9379) (-128.2585, -82.8802) (-127.9254, -82.8207) (-127.5929, -82.7594) (-127.2612, -82.6964) (-126.9301, -82.6315) (-126.5999, -82.5648) (-126.2703, -82.4962) (-125.9415, -82.4258) (-125.6136, -82.3535) (-125.2864, -82.2793) (-124.9601, -82.203) (-124.6347, -82.1248) (-124.3101, -82.0446) (-123.9864, -81.9623) (-123.6636, -81.8781) (-123.3417, -81.7919) (-123.0207, -81.7036) (-122.7007, -81.6132) (-122.3818, -81.5206) (-122.064, -81.4256) (-121.7473, -81.3283) (-121.4319, -81.2284) (-121.1176, -81.1262) (-120.8045, -81.0216) (-120.4924, -80.9149) (-120.1814, -80.8061) (-119.8715, -80.695) (-119.5629, -80.5814) (-119.256, -80.4646) (-118.951, -80.3443) (-118.6482, -80.2201) (-118.3475, -80.092) (-118.0487, -79.9606) (-117.7512, -79.8266) (-117.4549, -79.6908) (-117.1595, -79.5532) (-116.8657, -79.413) (-116.5749, -79.268) (-116.2887, -79.1151) (-116.0651, -78.9842) (-115.901, -78.8799) (-115.7932, -78.8076) (-115.7398, -78.7708) knots -1 -1 -1 -1 -1 -1 -0.98571429 -0.97142857 -0.95714286 -0.94285714 -0.92857143 -0.91428571 -0.9 -0.88571429 -0.87142857 -0.85714286 -0.84285714 -0.82857143 -0.81428571 -0.8 -0.78571429 -0.77142857 -0.75714286 -0.74285714 -0.72857143 -0.71428571 -0.7 -0.68571429 -0.67142857 -0.65714286 -0.64285714 -0.62857143 -0.61428571 -0.6 -0.58571429 -0.57142857 -0.55714286 -0.54285714 -0.52857143 -0.51428571 -0.5 -0.48571429 -0.47142857 -0.45714286 -0.44285714 -0.42857143 -0.41428571 -0.4 -0.38571429 -0.37142857 -0.35714286 -0.34285714 -0.32857143 -0.31428571 -0.3 -0.28571429 -0.27142857 -0.25714286 -0.24285714 -0.22857143 -0.21428571 -0.2 -0.18571429 -0.17142857 -0.15714286 -0.14285714 -0.12857143 -0.11428571 -0.1 -0.08571429 -0.07142857 -0.05714286 -0.04285714 -0.02857143 -0.01428571 0 0 0 0 0 0
  line L5 (-115.7398, -78.7708) -> (-112.0176, -76.2033)
  arc A11 (-109.82, -76.5937) -> (-112.0176, -76.2033) centre (-111.1163, -77.5101) ccw
  arc A12 (-109.82, -76.5937) -> (-103.2954, -85.0967) centre (2.1352, 2.5578) ccw
  arc A13 (-103.4871, -87.3205) -> (-103.2954, -85.0967) centre (-104.5161, -86.1116) ccw
  line L6 (-103.4871, -87.3205) -> (-106.9304, -90.2514)
  spline S6 degree 5 poles (-106.9304, -90.2514) (-106.9799, -90.2934) (-107.0776, -90.3788) (-107.2207, -90.5103) (-107.4052, -90.6924) (-107.6268, -90.9293) (-107.8422, -91.1727) (-108.0536, -91.4202) (-108.263, -91.6699) (-108.4709, -91.921) (-108.6773, -92.1736) (-108.8816, -92.4282) (-109.0832, -92.6855) (-109.2815, -92.9459) (-109.4767, -93.2093) (-109.6688, -93.4756) (-109.8585, -93.7442) (-110.046, -94.0148) (-110.2316, -94.287) (-110.4154, -94.5609) (-110.5975, -94.8363) (-110.7776, -95.1134) (-110.9556, -95.3922) (-111.1317, -95.6729) (-111.3056, -95.9553) (-111.4777, -96.2394) (-111.6478, -96.5251) (-111.8161, -96.8123) (-111.9827, -97.1009) (-112.1476, -97.3909) (-112.3108, -97.6823) (-112.4723, -97.975) (-112.6321, -98.2691) (-112.7902, -98.5646) (-112.9466, -98.8614) (-113.1014, -99.1595) (-113.2545, -99.4588) (-113.406, -99.7594) (-113.5559, -100.0612) (-113.7042, -100.3641) (-113.851, -100.6682) (-113.9962, -100.9735) (-114.1399, -101.2799) (-114.2821, -101.5875) (-114.4227, -101.8961) (-114.5618, -102.2058) (-114.6994, -102.5166) (-114.8355, -102.8285) (-114.9701, -103.1414) (-115.1033, -103.4553) (-115.235, -103.7702) (-115.3652, -104.0861) (-115.494, -104.403) (-115.6214, -104.7208) (-115.7473, -105.0396) (-115.8718, -105.3594) (-115.9949, -105.6801) (-116.1166, -106.0017) (-116.2368, -106.3242) (-116.3557, -106.6476) (-116.4732, -106.9719) (-116.5893, -107.297) (-116.704, -107.6231) (-116.8174, -107.95) (-116.9294, -108.2777) (-117.04, -108.6062) (-117.1493, -108.9356) (-117.2572, -109.2658) (-117.3638, -109.5968) (-117.469, -109.9286) (-117.5729, -110.2611) (-117.655, -110.5278) (-117.7159, -110.7282) (-117.7563, -110.8619) (-117.7764, -110.9288) knots 0 0 0 0 0 0 0.01428571 0.02857143 0.04285714 0.05714286 0.07142857 0.08571429 0.1 0.11428571 0.12857143 0.14285714 0.15714286 0.17142857 0.18571429 0.2 0.21428571 0.22857143 0.24285714 0.25714286 0.27142857 0.28571429 0.3 0.31428571 0.32857143 0.34285714 0.35714286 0.37142857 0.38571429 0.4 0.41428571 0.42857143 0.44285714 0.45714286 0.47142857 0.48571429 0.5 0.51428571 0.52857143 0.54285714 0.55714286 0.57142857 0.58571429 0.6 0.61428571 0.62857143 0.64285714 0.65714286 0.67142857 0.68571429 0.7 0.71428571 0.72857143 0.74285714 0.75714286 0.77142857 0.78571429 0.8 0.81428571 0.82857143 0.84285714 0.85714286 0.87142857 0.88571429 0.9 0.91428571 0.92857143 0.94285714 0.95714286 0.97142857 0.98571429 1 1 1 1 1 1
  arc A14 (-117.7764, -110.9288) -> (-111.3514, -117.3538) centre (2.1352, 2.5578) ccw
  spline S7 degree 5 poles (-111.3514, -117.3538) (-111.2845, -117.3337) (-111.1507, -117.2933) (-110.9504, -117.2324) (-110.6837, -117.1504) (-110.3511, -117.0464) (-110.0194, -116.9412) (-109.6884, -116.8346) (-109.3582, -116.7267) (-109.0288, -116.6174) (-108.7003, -116.5068) (-108.3725, -116.3948) (-108.0457, -116.2815) (-107.7196, -116.1667) (-107.3945, -116.0506) (-107.0702, -115.9331) (-106.7468, -115.8143) (-106.4243, -115.694) (-106.1027, -115.5723) (-105.782, -115.4492) (-105.4622, -115.3247) (-105.1434, -115.1988) (-104.8255, -115.0714) (-104.5087, -114.9426) (-104.1928, -114.8124) (-103.8778, -114.6807) (-103.5639, -114.5475) (-103.2511, -114.4129) (-102.9392, -114.2768) (-102.6284, -114.1392) (-102.3187, -114.0001) (-102.01, -113.8595) (-101.7025, -113.7173) (-101.3961, -113.5737) (-101.0908, -113.4284) (-100.7867, -113.2817) (-100.4837, -113.1333) (-100.182, -112.9834) (-99.8814, -112.8319) (-99.582, -112.6788) (-99.284, -112.524) (-98.9872, -112.3676) (-98.6917, -112.2096) (-98.3976, -112.0498) (-98.1049, -111.8883) (-97.8135, -111.725) (-97.5235, -111.5601) (-97.2349, -111.3935) (-96.9477, -111.2252) (-96.662, -111.0551) (-96.3779, -110.8831) (-96.0955, -110.7091) (-95.8148, -110.5331) (-95.5359, -110.355) (-95.2589, -110.1749) (-94.9834, -109.9929) (-94.7096, -109.809) (-94.4374, -109.6234) (-94.1668, -109.4359) (-93.8981, -109.2463) (-93.6319, -109.0541) (-93.3684, -108.8589) (-93.1081, -108.6606) (-92.8508, -108.459) (-92.5961, -108.2547) (-92.3435, -108.0484) (-92.0924, -107.8404) (-91.8428, -107.6311) (-91.5953, -107.4196) (-91.3518, -107.2043) (-91.115, -106.9826) (-90.9329, -106.7982) (-90.8013, -106.655) (-90.716, -106.5573) (-90.6739, -106.5079) knots -1 -1 -1 -1 -1 -1 -0.98571429 -0.97142857 -0.95714286 -0.94285714 -0.92857143 -0.91428571 -0.9 -0.88571429 -0.87142857 -0.85714286 -0.84285714 -0.82857143 -0.81428571 -0.8 -0.78571429 -0.77142857 -0.75714286 -0.74285714 -0.72857143 -0.71428571 -0.7 -0.68571429 -0.67142857 -0.65714286 -0.64285714 -0.62857143 -0.61428571 -0.6 -0.58571429 -0.57142857 -0.55714286 -0.54285714 -0.52857143 -0.51428571 -0.5 -0.48571429 -0.47142857 -0.45714286 -0.44285714 -0.42857143 -0.41428571 -0.4 -0.38571429 -0.37142857 -0.35714286 -0.34285714 -0.32857143 -0.31428571 -0.3 -0.28571429 -0.27142857 -0.25714286 -0.24285714 -0.22857143 -0.21428571 -0.2 -0.18571429 -0.17142857 -0.15714286 -0.14285714 -0.12857143 -0.11428571 -0.1 -0.08571429 -0.07142857 -0.05714286 -0.04285714 -0.02857143 -0.01428571 0 0 0 0 0 0
  line L7 (-90.6739, -106.5079) -> (-87.7431, -103.0646)
  arc A15 (-85.5193, -102.8728) -> (-87.7431, -103.0646) centre (-86.5342, -104.0935) ccw
  arc A16 (-85.5193, -102.8728) -> (-77.0163, -109.3974) centre (2.1352, 2.5578) ccw
  arc A17 (-76.6259, -111.5951) -> (-77.0163, -109.3974) centre (-77.9327, -110.6937) ccw
  line L8 (-76.6259, -111.5951) -> (-79.1933, -115.3172)
  spline S8 degree 5 poles (-79.1933, -115.3172) (-79.2302, -115.3707) (-79.3025, -115.4784) (-79.4067, -115.6425) (-79.5377, -115.8661) (-79.6905, -116.1523) (-79.8355, -116.4432) (-79.9758, -116.737) (-80.1134, -117.0323) (-80.2492, -117.3287) (-80.3832, -117.6261) (-80.5146, -117.9249) (-80.6427, -118.2256) (-80.7669, -118.5284) (-80.8872, -118.8334) (-81.004, -119.1403) (-81.1176, -119.4489) (-81.2287, -119.7588) (-81.3375, -120.0698) (-81.4442, -120.3819) (-81.5487, -120.695) (-81.651, -121.0093) (-81.7508, -121.3247) (-81.8482, -121.6414) (-81.9432, -121.9592) (-82.0358, -122.2782) (-82.1262, -122.5982) (-82.2144, -122.9191) (-82.3007, -123.241) (-82.3849, -123.5638) (-82.4671, -123.8875) (-82.5474, -124.2121) (-82.6256, -124.5375) (-82.7018, -124.8638) (-82.7761, -125.191) (-82.8484, -125.519) (-82.9188, -125.8477) (-82.9874, -126.1773) (-83.0541, -126.5076) (-83.1189, -126.8386) (-83.182, -127.1703) (-83.2433, -127.5028) (-83.3028, -127.836) (-83.3605, -128.1698) (-83.4164, -128.5043) (-83.4706, -128.8395) (-83.5231, -129.1753) (-83.5738, -129.5118) (-83.6229, -129.8488) (-83.6703, -130.1865) (-83.716, -130.5248) (-83.76, -130.8636) (-83.8024, -131.2031) (-83.8432, -131.543) (-83.8823, -131.8836) (-83.9198, -132.2247) (-83.9557, -132.5663) (-83.99, -132.9084) (-84.0227, -133.2511) (-84.0538, -133.5942) (-84.0834, -133.9379) (-84.1113, -134.282) (-84.1378, -134.6266) (-84.1627, -134.9717) (-84.186, -135.3172) (-84.2078, -135.6632) (-84.2281, -136.0097) (-84.2469, -136.3565) (-84.2642, -136.7038) (-84.28, -137.0515) (-84.2943, -137.3997) (-84.3045, -137.6785) (-84.3115, -137.8878) (-84.3159, -138.0274) (-84.318, -138.0973) knots 0 0 0 0 0 0 0.01428571 0.02857143 0.04285714 0.05714286 0.07142857 0.08571429 0.1 0.11428571 0.12857143 0.14285714 0.15714286 0.17142857 0.18571429 0.2 0.21428571 0.22857143 0.24285714 0.25714286 0.27142857 0.28571429 0.3 0.31428571 0.32857143 0.34285714 0.35714286 0.37142857 0.38571429 0.4 0.41428571 0.42857143 0.44285714 0.45714286 0.47142857 0.48571429 0.5 0.51428571 0.52857143 0.54285714 0.55714286 0.57142857 0.58571429 0.6 0.61428571 0.62857143 0.64285714 0.65714286 0.67142857 0.68571429 0.7 0.71428571 0.72857143 0.74285714 0.75714286 0.77142857 0.78571429 0.8 0.81428571 0.82857143 0.84285714 0.85714286 0.87142857 0.88571429 0.9 0.91428571 0.92857143 0.94285714 0.95714286 0.97142857 0.98571429 1 1 1 1 1 1
  arc A18 (-84.318, -138.0973) -> (-76.449, -142.6404) centre (2.1352, 2.5578) ccw
  spline S9 degree 5 poles (-76.449, -142.6404) (-76.3896, -142.6037) (-76.2709, -142.5301) (-76.0931, -142.4194) (-75.8567, -142.2711) (-75.5624, -142.0846) (-75.2692, -141.8971) (-74.977, -141.7085) (-74.686, -141.5188) (-74.3962, -141.328) (-74.1074, -141.1361) (-73.8199, -140.9431) (-73.5335, -140.749) (-73.2482, -140.5538) (-72.9642, -140.3575) (-72.6814, -140.1601) (-72.3998, -139.9616) (-72.1194, -139.7619) (-71.8402, -139.5611) (-71.5623, -139.3593) (-71.2857, -139.1562) (-71.0103, -138.9521) (-70.7363, -138.7468) (-70.4635, -138.5404) (-70.1921, -138.3328) (-69.922, -138.1241) (-69.6532, -137.9142) (-69.3859, -137.7032) (-69.1199, -137.491) (-68.8553, -137.2777) (-68.5921, -137.0631) (-68.3304, -136.8474) (-68.0701, -136.6305) (-67.8113, -136.4125) (-67.554, -136.1932) (-67.2983, -135.9727) (-67.044, -135.751) (-66.7913, -135.5281) (-66.5402, -135.3039) (-66.2907, -135.0786) (-66.0428, -134.8519) (-65.7966, -134.6241) (-65.5521, -134.3949) (-65.3094, -134.1644) (-65.0685, -133.9326) (-64.8293, -133.6996) (-64.5918, -133.4652) (-64.3562, -133.2296) (-64.1223, -132.9927) (-63.8904, -132.7544) (-63.6605, -132.5147) (-63.4327, -132.2736) (-63.2072, -132.0309) (-62.9839, -131.7867) (-62.7629, -131.5411) (-62.544, -131.294) (-62.327, -131.0455) (-62.1121, -130.7957) (-61.8992, -130.5446) (-61.6889, -130.2919) (-61.4814, -130.0373) (-61.2775, -129.7807) (-61.0773, -129.5217) (-60.8809, -129.2604) (-60.6879, -128.9972) (-60.4973, -128.7325) (-60.3085, -128.4666) (-60.1216, -128.1998) (-59.9373, -127.9315) (-59.7578, -127.6604) (-59.5864, -127.385) (-59.4582, -127.1598) (-59.3682, -126.9874) (-59.3111, -126.871) (-59.2833, -126.8123) knots -1 -1 -1 -1 -1 -1 -0.98571429 -0.97142857 -0.95714286 -0.94285714 -0.92857143 -0.91428571 -0.9 -0.88571429 -0.87142857 -0.85714286 -0.84285714 -0.82857143 -0.81428571 -0.8 -0.78571429 -0.77142857 -0.75714286 -0.74285714 -0.72857143 -0.71428571 -0.7 -0.68571429 -0.67142857 -0.65714286 -0.64285714 -0.62857143 -0.61428571 -0.6 -0.58571429 -0.57142857 -0.55714286 -0.54285714 -0.52857143 -0.51428571 -0.5 -0.48571429 -0.47142857 -0.45714286 -0.44285714 -0.42857143 -0.41428571 -0.4 -0.38571429 -0.37142857 -0.35714286 -0.34285714 -0.32857143 -0.31428571 -0.3 -0.28571429 -0.27142857 -0.25714286 -0.24285714 -0.22857143 -0.21428571 -0.2 -0.18571429 -0.17142857 -0.15714286 -0.14285714 -0.12857143 -0.11428571 -0.1 -0.08571429 -0.07142857 -0.05714286 -0.04285714 -0.02857143 -0.01428571 0 0 0 0 0 0
  line L9 (-59.2833, -126.8123) -> (-57.3435, -122.7278)
  arc A19 (-55.2451, -121.967) -> (-57.3435, -122.7278) centre (-55.9095, -123.4088) ccw
  arc A20 (-55.2451, -121.967) -> (-45.3431, -126.0686) centre (2.1352, 2.5578) ccw
  arc A21 (-44.3973, -128.0903) -> (-45.3431, -126.0686) centre (-45.8928, -127.5578) ccw
  line L10 (-44.3973, -128.0903) -> (-45.9138, -132.3501)
  spline S10 degree 5 poles (-45.9138, -132.3501) (-45.9356, -132.4113) (-45.9776, -132.534) (-46.0358, -132.7195) (-46.1044, -132.9694) (-46.178, -133.2854) (-46.2427, -133.6039) (-46.3021, -133.924) (-46.3586, -134.2449) (-46.4131, -134.5663) (-46.4656, -134.8882) (-46.5152, -135.2109) (-46.5611, -135.5345) (-46.6027, -135.8592) (-46.6399, -136.1849) (-46.6733, -136.5116) (-46.7032, -136.839) (-46.7303, -137.1671) (-46.7549, -137.4957) (-46.7772, -137.8248) (-46.7971, -138.1543) (-46.8145, -138.4843) (-46.8293, -138.8148) (-46.8414, -139.1459) (-46.8509, -139.4775) (-46.8578, -139.8095) (-46.8623, -140.142) (-46.8645, -140.4749) (-46.8644, -140.8082) (-46.8623, -141.1418) (-46.8579, -141.4757) (-46.8514, -141.81) (-46.8427, -142.1446) (-46.8319, -142.4795) (-46.819, -142.8147) (-46.804, -143.1502) (-46.7869, -143.486) (-46.7678, -143.8221) (-46.7467, -144.1584) (-46.7237, -144.4949) (-46.6988, -144.8317) (-46.6719, -145.1687) (-46.6431, -145.5059) (-46.6125, -145.8433) (-46.5799, -146.1809) (-46.5455, -146.5187) (-46.5093, -146.8566) (-46.4712, -147.1948) (-46.4314, -147.533) (-46.3898, -147.8715) (-46.3464, -148.21) (-46.3012, -148.5487) (-46.2543, -148.8876) (-46.2057, -149.2265) (-46.1553, -149.5656) (-46.1033, -149.9047) (-46.0495, -150.244) (-45.9941, -150.5834) (-45.937, -150.9228) (-45.8782, -151.2623) (-45.8178, -151.6019) (-45.7558, -151.9416) (-45.6922, -152.2813) (-45.6269, -152.621) (-45.56, -152.9608) (-45.4915, -153.3007) (-45.4215, -153.6406) (-45.3499, -153.9805) (-45.2767, -154.3204) (-45.2019, -154.6604) (-45.1256, -155.0003) (-45.0633, -155.2723) (-45.0159, -155.4763) (-44.984, -155.6123) (-44.968, -155.6803) knots 0 0 0 0 0 0 0.01428571 0.02857143 0.04285714 0.05714286 0.07142857 0.08571429 0.1 0.11428571 0.12857143 0.14285714 0.15714286 0.17142857 0.18571429 0.2 0.21428571 0.22857143 0.24285714 0.25714286 0.27142857 0.28571429 0.3 0.31428571 0.32857143 0.34285714 0.35714286 0.37142857 0.38571429 0.4 0.41428571 0.42857143 0.44285714 0.45714286 0.47142857 0.48571429 0.5 0.51428571 0.52857143 0.54285714 0.55714286 0.57142857 0.58571429 0.6 0.61428571 0.62857143 0.64285714 0.65714286 0.67142857 0.68571429 0.7 0.71428571 0.72857143 0.74285714 0.75714286 0.77142857 0.78571429 0.8 0.81428571 0.82857143 0.84285714 0.85714286 0.87142857 0.88571429 0.9 0.91428571 0.92857143 0.94285714 0.95714286 0.97142857 0.98571429 1 1 1 1 1 1
  arc A22 (-44.968, -155.6803) -> (-36.1913, -158.032) centre (2.1352, 2.5578) ccw
  spline S11 degree 5 poles (-36.1913, -158.032) (-36.1434, -157.9811) (-36.0477, -157.8793) (-35.9047, -157.7264) (-35.7148, -157.522) (-35.4787, -157.2657) (-35.244, -157.0087) (-35.0106, -156.7509) (-34.7786, -156.4923) (-34.548, -156.233) (-34.3188, -155.9729) (-34.091, -155.7121) (-33.8646, -155.4505) (-33.6396, -155.1881) (-33.416, -154.925) (-33.1939, -154.6611) (-32.9733, -154.3964) (-32.7541, -154.131) (-32.5365, -153.8648) (-32.3203, -153.5979) (-32.1056, -153.3302) (-31.8925, -153.0617) (-31.6809, -152.7925) (-31.4709, -152.5225) (-31.2624, -152.2518) (-31.0555, -151.9803) (-30.8503, -151.708) (-30.6466, -151.4349) (-30.4446, -151.1611) (-30.2442, -150.8866) (-30.0456, -150.6113) (-29.8486, -150.3352) (-29.6533, -150.0583) (-29.4598, -149.7807) (-29.268, -149.5023) (-29.078, -149.2231) (-28.8898, -148.9431) (-28.7035, -148.6624) (-28.5189, -148.3809) (-28.3362, -148.0986) (-28.1554, -147.8156) (-27.9766, -147.5317) (-27.7998, -147.2471) (-27.625, -146.9617) (-27.4522, -146.6754) (-27.2815, -146.3884) (-27.1128, -146.1006) (-26.9462, -145.812) (-26.7816, -145.5226) (-26.6192, -145.2324) (-26.4592, -144.9414) (-26.3016, -144.6495) (-26.1466, -144.3568) (-25.9941, -144.0631) (-25.8442, -143.7686) (-25.6967, -143.4733) (-25.5515, -143.1771) (-25.4085, -142.8803) (-25.2679, -142.5826) (-25.1301, -142.284) (-24.9956, -141.9845) (-24.865, -141.6837) (-24.7387, -141.3818) (-24.6166, -141.0786) (-24.4983, -140.7744) (-24.3827, -140.4693) (-24.2692, -140.1637) (-24.1577, -139.8576) (-24.0491, -139.5507) (-23.9459, -139.2425) (-23.8516, -138.9321) (-23.7861, -138.6813) (-23.7438, -138.4915) (-23.7188, -138.3643) (-23.707, -138.3004) knots -1 -1 -1 -1 -1 -1 -0.98571429 -0.97142857 -0.95714286 -0.94285714 -0.92857143 -0.91428571 -0.9 -0.88571429 -0.87142857 -0.85714286 -0.84285714 -0.82857143 -0.81428571 -0.8 -0.78571429 -0.77142857 -0.75714286 -0.74285714 -0.72857143 -0.71428571 -0.7 -0.68571429 -0.67142857 -0.65714286 -0.64285714 -0.62857143 -0.61428571 -0.6 -0.58571429 -0.57142857 -0.55714286 -0.54285714 -0.52857143 -0.51428571 -0.5 -0.48571429 -0.47142857 -0.45714286 -0.44285714 -0.42857143 -0.41428571 -0.4 -0.38571429 -0.37142857 -0.35714286 -0.34285714 -0.32857143 -0.31428571 -0.3 -0.28571429 -0.27142857 -0.25714286 -0.24285714 -0.22857143 -0.21428571 -0.2 -0.18571429 -0.17142857 -0.15714286 -0.14285714 -0.12857143 -0.11428571 -0.1 -0.08571429 -0.07142857 -0.05714286 -0.04285714 -0.02857143 -0.01428571 0 0 0 0 0 0
  line L11 (-23.707, -138.3004) -> (-22.8905, -133.853)
  arc A23 (-21.0605, -132.5751) -> (-22.8905, -133.853) centre (-21.3291, -134.1397) ccw
  arc A24 (-21.0605, -132.5751) -> (-10.4344, -133.974) centre (2.1352, 2.5578) ccw
  arc A25 (-8.9975, -135.6821) -> (-10.4344, -133.974) centre (-10.5799, -135.5548) ccw
  line L12 (-8.9975, -135.6821) -> (-9.3599, -140.1893)
  spline S12 degree 5 poles (-9.3599, -140.1893) (-9.3651, -140.254) (-9.3738, -140.3834) (-9.382, -140.5776) (-9.3837, -140.8368) (-9.3729, -141.161) (-9.3531, -141.4854) (-9.3276, -141.81) (-9.2991, -142.1346) (-9.2686, -142.4591) (-9.2359, -142.7837) (-9.2003, -143.1082) (-9.1609, -143.4326) (-9.117, -143.757) (-9.0687, -144.0813) (-9.0164, -144.4055) (-8.9605, -144.7295) (-8.9017, -145.0534) (-8.8405, -145.3772) (-8.7768, -145.7008) (-8.7108, -146.0243) (-8.6422, -146.3475) (-8.571, -146.6706) (-8.497, -146.9936) (-8.4203, -147.3163) (-8.341, -147.6388) (-8.2593, -147.9611) (-8.1753, -148.2833) (-8.089, -148.6051) (-8.0005, -148.9268) (-7.9099, -149.2482) (-7.8171, -149.5694) (-7.7221, -149.8904) (-7.625, -150.2111) (-7.5257, -150.5315) (-7.4244, -150.8517) (-7.321, -151.1717) (-7.2156, -151.4913) (-7.1082, -151.8107) (-6.9989, -152.1299) (-6.8876, -152.4487) (-6.7744, -152.7672) (-6.6594, -153.0855) (-6.5424, -153.4035) (-6.4236, -153.7211) (-6.3029, -154.0385) (-6.1805, -154.3556) (-6.0562, -154.6723) (-5.9302, -154.9888) (-5.8024, -155.3049) (-5.6728, -155.6207) (-5.5415, -155.9362) (-5.4085, -156.2513) (-5.2738, -156.5661) (-5.1374, -156.8806) (-4.9994, -157.1947) (-4.8596, -157.5085) (-4.7183, -157.822) (-4.5753, -158.1351) (-4.4306, -158.4478) (-4.2844, -158.7602) (-4.1366, -159.0722) (-3.9872, -159.3839) (-3.8362, -159.6952) (-3.6836, -160.0061) (-3.5295, -160.3167) (-3.3739, -160.6268) (-3.2167, -160.9366) (-3.0581, -161.246) (-2.8979, -161.555) (-2.7362, -161.8637) (-2.6056, -162.1103) (-2.5071, -162.295) (-2.441, -162.4181) (-2.4079, -162.4797) knots 0 0 0 0 0 0 0.01428571 0.02857143 0.04285714 0.05714286 0.07142857 0.08571429 0.1 0.11428571 0.12857143 0.14285714 0.15714286 0.17142857 0.18571429 0.2 0.21428571 0.22857143 0.24285714 0.25714286 0.27142857 0.28571429 0.3 0.31428571 0.32857143 0.34285714 0.35714286 0.37142857 0.38571429 0.4 0.41428571 0.42857143 0.44285714 0.45714286 0.47142857 0.48571429 0.5 0.51428571 0.52857143 0.54285714 0.55714286 0.57142857 0.58571429 0.6 0.61428571 0.62857143 0.64285714 0.65714286 0.67142857 0.68571429 0.7 0.71428571 0.72857143 0.74285714 0.75714286 0.77142857 0.78571429 0.8 0.81428571 0.82857143 0.84285714 0.85714286 0.87142857 0.88571429 0.9 0.91428571 0.92857143 0.94285714 0.95714286 0.97142857 0.98571429 1 1 1 1 1 1
  arc A26 (-2.4079, -162.4797) -> (6.6784, -162.4797) centre (2.1352, 2.5578) ccw